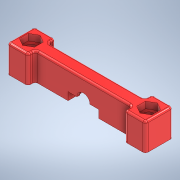
# Autodesk Inventor part: Mancal superior
Saved by Autodesk Inventor 2021 (Build 250183000, 183)
## iProperties
Created: 2021-11-16
Part Number: Mancal superior
Material: Generic
Document SubType Name: Modeling
Designer: Matheus
Density: 0.700696 g/cm^3
Appearance: Default
Mass: 2.2 g
Surface Area: 22.6154 cm^2
Volume: 3.13973 cm^3
Author: Mathe
Autodesk Inventor part; units mm, degrees
ref_plane "YZ Plane" through (0, 0, 0) normal (1, 0, 0) x (0, 1, 0)
ref_plane "XZ Plane" through (0, 0, 0) normal (0, 1, 0) x (-1, 0, 0)
ref_plane "XY Plane" through (0, 0, 0) normal (0, 0, 1) x (1, 0, 0)
sketch "Sketch1" plane through (0, 0, 0) normal (0, 0, 1) x (1, 0, 0)
  line L0 (-37.1, 0) -> (37.1, 0) construction
  line L1 (0, 12.6) -> (0, -2.1) construction
  line L2 (26.5, 10.5) -> (26.5, 0)
  line L3 (26.5, 10.5) -> (-26.5, 10.5)
  line L4 (-26.5, 10.5) -> (-26.5, 0)
  arc A0 (2.5, 3) -> (-2.5, 3) centre (0, 3) ccw
  line L5 (-26.5, 0) -> (-5.9, 0)
  line L6 (5.9, 0) -> (26.5, 0)
  line L7 (-5.9, 0) -> (-5.9, 3)
  line L8 (-5.9, 3) -> (-2.5, 3)
  line L9 (2.5, 3) -> (5.9, 3)
  line L10 (5.9, 3) -> (5.9, 0)
  point P0 (0, 0)
  dimension "d1" = 10.5
  dimension "d2" = 2.5
  dimension "d4" = 53
  dimension "d5" = 11.8
  dimension "d23" = 3
  constraints: 18 end point, 6 point on line, 4 perpendicular, 2 collinear, 2 point on circle, 1 centre point, 1 horizontal, 1 vertical, 2 other
  measures "d1" distance between parallel lines of L0 L3
  measures "d2" radius of A0
  measures "d4" distance between parallel lines of L2 L4
  measures "d5" distance between parallel lines of L10 L7
  measures "d23" distance between parallel lines of L0 L8
extrude "Extrusion1" add sketch "Sketch1" along normal mid plane 5
sketch "Sketch2" plane through (0, 0, 0) normal (0, 0, 1) x (1, 0, 0)
  arc A0 (2.5, 3) -> (-2.5, 3) centre (0, 3) ccw construction
  line L0 (0, 7.41) -> (0, -1.41) construction
  circle A1 centre (0, 3) radius 3.15
  point P0 (0, 0)
  dimension "d9" = 6.3
  constraints: 1 centre point, 1 coincident
  measures "d9" diameter of A1
extrude "Extrusion2" cut sketch "Sketch2" along normal mid plane 2.8
sketch "Sketch4" plane through (-26.5, 10.5, 2.5) normal (0, 1, 0) x (1, 0, 0)
  line L0 (0, -2.75) -> (8, -2.75)
  line L1 (8, -2.75) -> (8, 7.75)
  line L2 (8, 7.75) -> (0, 7.75)
  line L3 (0, 7.75) -> (0, -2.75)
  line L4 (63.6, 2.5) -> (-10.6, 2.5) construction
  line L5 (26.5, 9.85) -> (26.5, -4.85) construction
  line L6 (0, 5) -> (0, 0) construction
  line L7 (53, -2.75) -> (45, -2.75)
  line L8 (45, -2.75) -> (45, 7.75)
  line L9 (45, 7.75) -> (53, 7.75)
  line L10 (53, 7.75) -> (53, -2.75)
  line L11 (53, 5) -> (53, 0) construction
  line L12 (49, -2.75) -> (49, 7.75) construction
  line L13 (4, -2.75) -> (4, 7.75) construction
  point P0 (26.5, 2.5)
  point P1 (4, 2.5)
  point P2 (49, 2.5)
  dimension "d24" = 8
  dimension "d25" = 10.5
  constraints: 22 end point, 6 midpoint, 6 symmetric about line, 2 parallel, 2 point on line, 1 collinear, 1 horizontal, 1 perpendicular, 1 other
  measures "d24" distance between parallel lines of L1 L3
  measures "d25" distance between parallel lines of L2 L0
extrude "Extrusion4" add sketch "Sketch4" against normal up to surface (10.5 mm away)
hole "Hole1" at (-22.5, 10.5, 0) at (22.5, 10.5, 0) direction (0, -1, 0) diameter 3.5 depth 10.5
sketch "Sketch5" plane through (-26.5, 10.5, -5.25) normal (0, 1, 0) x (1, 0, 0)
  circle A0 centre (4, -5.25) radius 1.75 construction
  line L0 (1.1, -3.5757) -> (4, -1.9014)
  line L1 (4, -1.9014) -> (6.9, -3.5757)
  line L2 (6.9, -3.5757) -> (6.9, -6.9243)
  line L3 (6.9, -6.9243) -> (4, -8.5986)
  line L4 (4, -8.5986) -> (1.1, -6.9243)
  line L5 (1.1, -6.9243) -> (1.1, -3.5757)
  line L6 (26.5, 2.1) -> (26.5, -12.6) construction
  circle A1 centre (49, -5.25) radius 1.75 construction
  line L7 (51.9, -3.5757) -> (49, -1.9014)
  line L8 (49, -1.9014) -> (46.1, -3.5757)
  line L9 (46.1, -3.5757) -> (46.1, -6.9243)
  line L10 (46.1, -6.9243) -> (49, -8.5986)
  line L11 (49, -8.5986) -> (51.9, -6.9243)
  line L12 (51.9, -6.9243) -> (51.9, -3.5757)
  point P0 (26.5, -5.25)
  dimension "d35" = 5.8
  constraints: 24 end point, 8 symmetric about line, 2 coincident, 1 centre point, 1 vertical, 14 other
  measures "d35" distance between parallel lines of L2 L5
extrude "Extrusion5" cut sketch "Sketch5" against normal blind 2.5
fillet "Fillet3" radius 1 12 edges at (-18.5, 5.25, 2.5) (-18.5, 5.25, 5.25) (18.5, 5.25, 2.5) (18.5, 5.25, 5.25) (26.5, 5.25, 5.25) (26.5, 5.25, -5.25) (18.5, 5.25, -5.25) (18.5, 5.25, -2.5) (-18.5, 5.25, -2.5) (-18.5, 5.25, -5.25) (-26.5, 5.25, -5.25) (-26.5, 5.25, 5.25)
fillet "Fillet4" radius 0.75 24 edges at (-18.2071, 10.5, 2.7929) (-18.5, 10.5, 3.875) (-18.7929, 10.5, 4.9571) (-22.5, 10.5, 5.25) (-26.2071, 10.5, 4.9571) (-26.5, 10.5, 0) (-26.2071, 10.5, -4.9571) (-22.5, 10.5, -5.25) (-18.7929, 10.5, -4.9571) (-18.5, 10.5, -3.875) (-18.2071, 10.5, -2.7929) (0, 10.5, -2.5) (18.2071, 10.5, -2.7929) (18.5, 10.5, -3.875) (18.7929, 10.5, -4.9571) (22.5, 10.5, -5.25) (26.2071, 10.5, -4.9571) (26.5, 10.5, 0) (26.2071, 10.5, 4.9571) (22.5, 10.5, 5.25) (18.7929, 10.5, 4.9571) (18.5, 10.5, 3.875) (18.2071, 10.5, 2.7929) (0, 10.5, 2.5)
body "Solid1"
